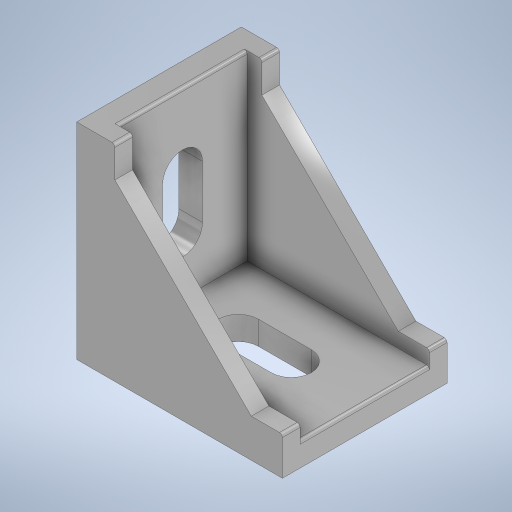
# Autodesk Inventor part: L Angle Bracket 30x30 31082023
Saved by Autodesk Inventor 2024 (Build 280153000, 153)
## iProperties
Created: 2023-08-31
Part Number: L Angle Bracket 30x30 31082023
Material: Generic
Document SubType Name: Modeling
Designer: Marcel
Density: 1 g/cm^3
Appearance: Aluminum - Polished
Author: Marcel
Autodesk Inventor part; units mm, degrees
ref_plane "YZ Plane" through (0, 0, 0) normal (1, 0, 0) x (0, 1, 0)
sketch "Sketch1" plane through (0, 0, 0) normal (0, 0, 1) x (1, 0, 0)
  line L0 (0, 0) -> (0, 35)
  line L1 (0, 35) -> (4, 35)
  line L2 (4, 35) -> (4, 4)
  line L3 (4, 4) -> (35, 4)
  line L4 (35, 4) -> (35, 0)
  line L5 (35, 0) -> (0, 0)
  dimension "d8" = 35
  dimension "d10" = 4
  dimension "d11" = 4
  dimension "d12" = 35
  constraints: 12 end point, 5 perpendicular, 1 vertical
  measures "d8" distance of L0.start L0.end
  measures "d10" distance between parallel lines of L0 L2
  measures "d11" distance between parallel lines of L5 L3
  measures "d12" distance of L4.end L0.start
extrude "Extrusion1" add sketch "Sketch1" along normal blind 11 and the other way blind 11
ref_plane "Work Plane1" through (0, 0, -11) normal (-0.7071, 0.7071, 0) x (0, 0, -1)
sketch "Sketch2" plane through (4, 4, -11) normal (1, 0, 0) x (0, 0, -1)
  line L0 (-11, 21.9) -> (-11, 6.1) construction
  line L1 (-14.4, 18.5) -> (-14.4, 9.5)
  line L2 (-7.6, 9.5) -> (-7.6, 18.5)
  arc A0 (-7.6, 18.5) -> (-14.4, 18.5) centre (-11, 18.5) ccw
  arc A1 (-14.4, 9.5) -> (-7.6, 9.5) centre (-11, 9.5) ccw
  line L3 (0, 0) -> (-22, 0) projected
  line L4 (-22, -4) -> (-11, -4) projected
  line L5 (-22, 0) -> (-22, 31) projected
  point P0 (-11, 14)
  dimension "d16" = 6.8
  dimension "d17" = 9
  dimension "d19" = 13.5
  dimension "d28" = 11
  constraints: 8 end point, 6 point on circle, 4 tangent, 2 centre point, 2 point on line, 1 midpoint, 1 parallel, 1 vertical
  measures "d16" diameter of A1
  measures "d17" distance of A1.centre A0.centre
  measures "d19" distance from line of A1.centre L4
  measures "d28" distance from line of L5 A0.centre
extrude "Extrusion2" cut sketch "Sketch2" against normal up to surface (4 mm away)
mirror "Mirror1" about plane through (0, 0, -11) normal (-0.7071, 0.7071, 0) of "Extrusion2"
sketch "Sketch3" plane through (0, 0, 11) normal (0, 0, 1) x (1, 0, 0)
  line L0 (4, 35) -> (0, 35) projected
  line L1 (0, 35) -> (6.5, 35)
  line L2 (6.5, 35) -> (6.5, 29.7)
  line L3 (35, 0) -> (35, 4) projected
  line L4 (35, 0) -> (35, 6.5)
  line L5 (35, 6.5) -> (29.7, 6.5)
  line L6 (29.7, 6.5) -> (6.5, 29.7)
  line L7 (0, 35) -> (0, 0) projected
  line L8 (0, 35) -> (0, 0)
  line L9 (0, 0) -> (35, 0)
  dimension "d22" = 6.5
  dimension "d23" = 5.3
  dimension "d24" = 6.5
  dimension "d25" = 5.3
  constraints: 14 end point, 3 perpendicular, 2 collinear, 1 vertical
  measures "d22" distance of L0.end L1.end
  measures "d23" distance of L1.end L2.end
  measures "d24" distance of L3.start L4.end
  measures "d25" distance of L4.end L5.end
ref_plane "Work Plane2" through (0, 0, 0) normal (0, 0, 1) x (1, 0, 0)
extrude "Extrusion3" add sketch "Sketch3" along normal blind 3
mirror "Mirror2" about plane through (0, 0, 0) normal (0, 0, 1) of "Extrusion3"
fillet "Fillet1" radius 0.5 6 edges at (35, 6.5, 12.5) (35, 6.5, -12.5) (6.5, 35, -12.5) (6.5, 35, 12.5) (35, 4, 0) (4, 35, 0)
sketch "Sketch4" plane through (0, 0, 14) normal (0, -1, 0) x (1, 0, 0)
  line L0 (35, -3) -> (35, -25) projected
  line L1 (35, -14) -> (0, -14) construction
  line L2 (4.5, -11.2) -> (2.5, -11.2)
  line L3 (2.5, -11.2) -> (2.5, -16.8)
  line L4 (2.5, -16.8) -> (4.5, -16.8)
  line L5 (4.5, -16.8) -> (4.5, -11.2)
  line L6 (4.5, -11.2) -> (2.5, -16.8) construction
  line L7 (2.5, -11.2) -> (4.5, -16.8) construction
  line L8 (0, -28) -> (0, 0) projected
  line L9 (30.5, -11.2) -> (32.5, -11.2)
  line L10 (32.5, -11.2) -> (32.5, -16.8)
  line L11 (32.5, -16.8) -> (30.5, -16.8)
  line L12 (30.5, -16.8) -> (30.5, -11.2)
  line L13 (30.5, -11.2) -> (32.5, -16.8) construction
  line L14 (32.5, -11.2) -> (30.5, -16.8) construction
  point P0 (3.5, -14)
  point P1 (31.5, -14)
  dimension "d34" = 2
  dimension "d35" = 5.6
  dimension "d36" = 2.5
  dimension "d37" = 5.6
  dimension "d38" = 2
  dimension "d39" = 2.5
  constraints: 26 end point, 5 midpoint, 4 parallel, 3 horizontal, 2 perpendicular, 2 point on line
  measures "d34" distance of L3.end L4.end
  measures "d35" distance of L4.end L2.start
  measures "d36" distance between parallel lines of L8 L3
  measures "d37" distance of L9.end L10.end
  measures "d38" distance of L10.end L11.end
  measures "d39" distance between parallel lines of L10 L0
extrude "Extrusion4" add sketch "Sketch4" along normal blind 2
mirror "Mirror3" about plane through (0, 0, -11) normal (-0.7071, 0.7071, 0) of "Extrusion4"
body "Solid1"
